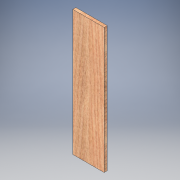
# Autodesk Inventor part: support1
Saved by Autodesk Inventor 2019 (Build 230136000, 136)
## iProperties
Created: 2019-01-07
Part Number: support1
Material: Wood (Birch)
Document SubType Name: Modeling
Designer: gaincarlo
Density: 0.55 g/cm^3
Appearance: Birch - Natural Polished
Author: gaincarlo
Autodesk Inventor part; units mm, degrees
ref_plane "YZ Plane" through (0, 0, 0) normal (1, 0, 0) x (0, 1, 0)
ref_plane "XZ Plane" through (0, 0, 0) normal (0, 1, 0) x (-1, 0, 0)
ref_plane "Work Plane1" through (0, 0, 0) normal (0, 0, 1) x (1, 0, 0)
sketch "Sketch1" plane through (0, 0, 0) normal (0, 0, 1) x (1, 0, 0)
  line L0 (0, 0) -> (0, 3) construction
  line L1 (0, 3) -> (217.415, 3) construction
  line L2 (217.415, 3) -> (217.415, 0) construction
  line L3 (217.415, 0) -> (0, 0) construction
  line L4 (217.415, 0) -> (117.415, 0)
  line L5 (117.415, 0) -> (117.415, 400)
  line L6 (117.415, 400) -> (217.415, 400)
  line L7 (217.415, 400) -> (217.415, 0)
  dimension "d0" = 100
  dimension "d1" = 400
  constraints: 16 end point, 3 horizontal, 2 parallel, 2 vertical, 1 perpendicular, 3 other
  measures "d0" distance of L5.end L6.end
  measures "d1" distance of L4.end L5.end
extrude "Extrusion1" add sketch "Sketch1" along normal blind 10
body "Solid1"
